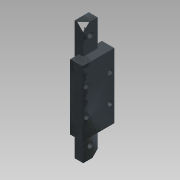
# Autodesk Inventor part: 90_Linearführung
Saved by Autodesk Inventor 2015 (Build 190159000, 159)
## iProperties
Created: 2016-03-16
Part Number: 90_Linearführung
Material: Eisen, grau
Document SubType Name: Modeling
Designer: Bene
Density: 7.15 g/cm^3
Appearance: Eisen - grau
Author: Bene
Autodesk Inventor part; units mm, degrees
ref_plane "YZ Plane" through (0, 0, 0) normal (1, 0, 0) x (0, 1, 0)
ref_plane "XZ Plane" through (0, 0, 0) normal (0, 1, 0) x (-1, 0, 0)
ref_plane "XY Plane" through (0, 0, 0) normal (0, 0, 1) x (1, 0, 0)
sketch "Skizze1" plane through (0, 0, 0) normal (1, 0, 0) x (0, 1, 0)
  line L0 (0, 0) -> (9, 0)
  line L1 (9, 0) -> (9, 75)
  line L2 (9, 75) -> (0, 75)
  line L3 (0, 75) -> (0, 0)
  dimension "d0" = 9
  dimension "d1" = 75
  constraints: 8 end point, 2 parallel, 1 horizontal, 1 perpendicular
  measures "d0" distance of L2.end L1.end
  measures "d1" distance of L1.end L0.end
extrude "Extrusion1" add sketch "Skizze1" along normal blind 5.5
sketch "Skizze2" plane through (5.5, 0, 0) normal (1, 0, 0) x (0, 0, -1)
  line L0 (0, 0) -> (0, 9) projected
  line L1 (0, 9) -> (-75, 9) projected
  line L2 (-75, 9) -> (-75, 0) projected
  line L3 (-75, 0) -> (0, 0) projected
  circle A0 centre (-67.5, 4.5) radius 1.75
  circle A1 centre (-7.5, 4.5) radius 1.75
  circle A2 centre (-47.5, 4.5) radius 1.75
  circle A3 centre (-27.5, 4.5) radius 1.75
  dimension "d4" = 3.5
  dimension "d5" = 7.5
  dimension "d6" = 3.5
  dimension "d7" = 7.5
  dimension "d8" = 3.5
  dimension "d9" = 20
  dimension "d10" = 3.5
  dimension "d11" = 20
  constraints: 4 centre point
  measures "d4" diameter of A0
  measures "d5" distance from line of L2 A0.centre
  measures "d6" diameter of A1
  measures "d7" distance from line of A1.centre L0
  measures "d8" diameter of A2
  measures "d9" distance of A2.centre A0.centre
  measures "d10" diameter of A3
  measures "d11" distance of A3.centre A1.centre
extrude "Extrusion2" cut sketch "Skizze2" against normal through all contours A0 | A1 | A2 | A3
sketch "Skizze3" plane through (5.5, 0, 0) normal (1, 0, 0) x (0, 0, -1)
  circle A0 centre (-47.5, 4.5) radius 1.75 projected
  circle A1 centre (-67.5, 4.5) radius 1.75 projected
  circle A2 centre (-7.5, 4.5) radius 1.75 projected
  circle A3 centre (-27.5, 4.5) radius 1.75 projected
  line L0 (0, 0) -> (0, 9) projected
  line L1 (0, 9) -> (-75, 9) projected
  line L2 (-75, 9) -> (-75, 0) projected
  line L3 (-75, 0) -> (0, 0) projected
  line L4 (-58, 14.5) -> (-17, 14.5)
  line L5 (-17, 14.5) -> (-17, -5.5)
  line L6 (-17, -5.5) -> (-58, -5.5)
  line L7 (-58, -5.5) -> (-58, 14.5)
  line L8 (-58, 14.5) -> (-17, -5.5) construction
  line L9 (-17, 14.5) -> (-58, -5.5) construction
  point P0 (-37.5, 4.5)
  dimension "d15" = 41
  dimension "d16" = 20
  constraints: 12 end point, 2 midpoint, 2 parallel, 1 horizontal, 1 perpendicular
  measures "d15" distance of L5.end L6.end
  measures "d16" distance of L4.end L5.end
extrude "Extrusion3" add sketch "Skizze3" along normal blind 5 and the other way blind 2.75 contours A0 | A3 | L5 L6 L7 L3 | L3 L7 L1 L5 | L1 L7 L4 L5
sketch "Skizze4" plane through (10.5, 0, 0) normal (1, 0, 0) x (0, 0, -1)
  line L0 (-17, 14.5) -> (-58, 14.5) projected
  line L1 (-58, 14.5) -> (-58, -5.5) projected
  line L2 (-58, -5.5) -> (-17, -5.5) projected
  line L3 (-17, -5.5) -> (-17, 14.5) projected
  circle A0 centre (-46, -3) radius 1.5
  circle A1 centre (-46, 12) radius 1.5
  circle A2 centre (-29, -2.75) radius 1.5
  circle A3 centre (-29, 12) radius 1.5
  circle A4 centre (-29, -2.75) radius 1.5 projected
  circle A5 centre (-29, 12) radius 1.5 projected
  circle A6 centre (-46, 12) radius 1.5 projected
  circle A7 centre (-46, -3) radius 1.5 projected
  line L4 (-23, -4.9525) -> (-23, 23.5) projected
  line L5 (-23, 23.5) -> (-58, 23.5) projected
  line L6 (-58, 23.5) -> (-58, -4.9525) projected
  line L7 (-23, -4.9525) -> (-58, -4.9525) projected
  circle A8 centre (-46, 21.0354) radius 1.5
  circle A9 centre (-30.5, 21.0354) radius 1.5
  circle A10 centre (-46, 20.5472) radius 1.5 projected
  circle A11 centre (-30.5, 20.5472) radius 1.5 projected
  point P0 (0, 0)
  dimension "d21" = 3
  dimension "d22" = 3
  dimension "d23" = 3
  dimension "d24" = 3
  dimension "d27" = 3
  dimension "d28" = 3
  constraints: 6 centre point
  measures "d21" diameter of A0
  measures "d22" diameter of A1
  measures "d23" diameter of A2
  measures "d24" diameter of A3
  measures "d27" diameter of A8
  measures "d28" diameter of A9
extrude "Extrusion4" cut sketch "Skizze4" against normal blind 5 contours A0 | A1 | A2 | A3 | A8 A10 | A10 A8 | A9 A11 | A11 A9 picked at (-46.157, 22.1946) picked at (-45.8838, 21.1962) picked at (-30.657, 22.1946) picked at (-30.3838, 20.3864)
